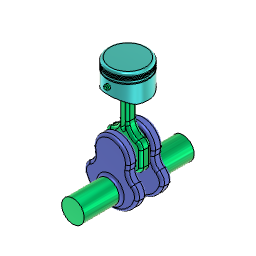
piston v2 (Autodesk Fusion 360 design; units mm, degrees)
Autodesk Fusion 360 part; units mm, degrees
sketch "Sketch1" plane through (0, 0, 0) normal (0, 0, 1) x (1, 0, 0) in component "Component"
  line L0 (100, 57.735) -> (0, 115.4701)
  line L1 (0, 115.4701) -> (-100, 57.735)
  line L2 (-100, 57.735) -> (-100, -57.735)
  line L3 (-100, -57.735) -> (0, -115.4701)
  line L4 (0, -115.4701) -> (100, -57.735)
  line L5 (100, -57.735) -> (100, 57.735)
  circle A0 centre (0, 0) radius 60
  constraint coincident A0.centre origin
extrude "Extrude1" add sketch "Sketch1" against normal blind 70 contours L0 L1 L2 L3 L4 L5 | A0 makes body 1 in component "Component"
extrude "Extrude2" add sketch "Sketch1" along normal blind 325 contours A0 bodies 1 in component "Component"
thread "Thread1" "ISO Metric profile 120.0 M120x6 6g" major diameter 119.62 minor diameter 112.7258 pitch 6 angle 60 resizes the face on face at (59.7018, -5.9741, 108.3333) from (0, 0, 75) to (0, 0, 325) on bodies 1 in component "Component"
sketch "Sketch1 (2)" plane through (0, 0, 0) normal (0, 1, 0) x (1, 0, 0) in component "piston"
  line L0 (0, -84) -> (0, -139)
  line L1 (0, -139) -> (40, -139)
  line L2 (40, -139) -> (40, -132)
  line L3 (40, -132) -> (36, -132)
  line L4 (36, -132) -> (36, -130)
  line L5 (36, -130) -> (40, -130)
  line L6 (40, -130) -> (40, -128)
  line L7 (40, -128) -> (36, -128)
  line L8 (36, -128) -> (36, -126)
  line L9 (36, -126) -> (40, -126)
  line L10 (40, -126) -> (40, -122)
  line L11 (40, -122) -> (36, -122)
  line L12 (36, -122) -> (36, -120)
  line L13 (36, -120) -> (40, -120)
  line L14 (40, -120) -> (40, -84)
  line L15 (40, -84) -> (0, -84)
  dimension "d7" = 40
  dimension "d8" = 4
  dimension "d9" = 4
  dimension "d10" = 7
  dimension "d11" = 2
  dimension "d12" = 2
  dimension "d13" = 2
  dimension "d14" = 4
  dimension "d15" = 2
  dimension "d16" = 36
  constraint vertical L0
  constraint perpendicular L0 L1
  constraint perpendicular L1 L2
  constraint perpendicular L2 L3
  constraint perpendicular L3 L4
  constraint perpendicular L4 L5
  constraint perpendicular L5 L6
  constraint perpendicular L6 L7
  constraint perpendicular L7 L8
  constraint perpendicular L6 L9
  constraint perpendicular L9 L10
  constraint perpendicular L10 L11
  constraint perpendicular L11 L12
  constraint perpendicular L12 L13
  constraint perpendicular L13 L14
  constraint perpendicular L0 L15
  constraint equal L3 L5
  constraint equal L5 L7
  constraint equal L7 L9
  constraint equal L11 L13
  measures "d7" distance of L0.end L1.end
  measures "d8" distance of L2.end L3.end
  measures "d9" distance of L10.end L11.end
  measures "d10" distance of L1.end L2.end
  measures "d11" distance of L3.end L4.end
  measures "d12" distance of L5.end L6.end
  measures "d13" distance of L7.end L8.end
  measures "d14" distance of L9.end L10.end
  measures "d15" distance of L11.end L12.end
  measures "d16" distance of L13.end L14.end
revolve "Revolve1" add sketch "Sketch1 (2)" angle 360 about axis through (0, 0, 1.75) along (0, 0, 1) separate body makes body 2 in component "piston"
move_body "Move1" bodies 2 to x (1, 0, 0) y (0, 1, 0) z (0, 0, 1) at (0, 0, -44) in component "piston"
sketch "Sketch2" plane through (0, 0, 0) normal (0, 1, 0) x (1, 0, 0) in component "piston"
  line L0 (0, 0) -> (0, -143.3697)
  line L1 (-40, -40) -> (40, -40)
  arc A0 (-35.5, -40) -> (35.5, -40) centre (0, 18.0125) ccw
  line L2 (-35.5, 0) -> (35.5, 0)
  line L3 (35.5, 0) -> (35.5, -40)
  line L4 (-35.5, -40) -> (-35.5, -36.7221)
  line L5 (-35.5, -36.7221) -> (-35.5, 0)
  point P0 (0, -50)
  point P1 (35.5, -40)
  point P2 (-35.5, -40)
  dimension "d18" = 10
  dimension "d19" = 4.5
  dimension "d20" = 4.5
  constraint coincident L0.start origin
  constraint vertical L0
  constraint coincident L0 P0
  constraint coincident L1 P1
  constraint coincident L1 P2
  constraint coincident P0 A0
  constraint coincident P1 A0.end
  constraint coincident P2 A0.start
  constraint perpendicular L0 L2
  constraint vertical L3
  constraint perpendicular L1 L4
  constraint perpendicular L2 L5
  measures "d18" distance of P0 L1
  measures "d19" distance of L1.end P1
  measures "d20" distance of L1.start P2
sketch "Sketch3" plane through (0, 0, 40) normal (0, 0, -1) x (1, 0, 0) in component "piston"
  circle A0 centre (0, 0) radius 40
  circle A1 centre (0, 0) radius 35.5
  dimension "d21" = 71
  constraint coincident A0.centre A1.centre
  measures "d21" diameter of A1
extrude "Extrude1'" cut sketch "Sketch3" against normal blind 33 contours A1 bodies 2 in component "piston"
extrude "Extrude2'" cut sketch "Sketch2" along normal mid plane 100 bodies 2 in component "piston"
sketch "Sketch4" plane through (0, 0, 0) normal (0, 1, 0) x (1, 0, 0) in component "piston"
  circle A0 centre (0, -64) radius 5
  line L0 (35.5, -40) -> (40, -40)
  dimension "d26" = 24
  measures "d26" distance of A0.centre L0
extrude "Extrude3" cut sketch "Sketch4" along normal mid plane 140 bodies 2 in component "piston"
sketch "Sketch5" plane through (0, 0, 0) normal (0, 1, 0) x (1, 0, 0) in component "piston"
  spline S0 degree 3 poles (-5, -64) (-5, -64.6285) (-4.8743, -65.2985) (-4.3638, -66.5302) (-3.9791, -67.092) (-3.092, -67.9791) (-2.5302, -68.3638) (-1.2985, -68.8743) (-0.6285, -69) (0.6285, -69) (1.2985, -68.8743) (2.5302, -68.3638) (3.092, -67.9791) (3.9791, -67.092) (4.3638, -66.5302) (4.8743, -65.2985) (5, -64.6285) (5, -63.3715) (4.8743, -62.7015) (4.3638, -61.4698) (3.9791, -60.908) (3.092, -60.0209) (2.5302, -59.6362) (1.2985, -59.1257) (0.6285, -59) (-0.6285, -59) (-1.2985, -59.1257) (-2.5302, -59.6362) (-3.092, -60.0209) (-3.9791, -60.908) (-4.3638, -61.4698) (-4.8743, -62.7015) (-5, -63.3715) (-5, -64) knots 0 0 0 0 0.188556 0.188556 0.377112 0.377112 0.565667 0.565667 0.754221 0.754221 0.942775 0.942775 1.13133 1.13133 1.319886 1.319886 1.508442 1.508442 1.696998 1.696998 1.885554 1.885554 2.074108 2.074108 2.262663 2.262663 2.451217 2.451217 2.639772 2.639772 2.828328 2.828328 3.016884 3.016884 3.016884 3.016884
  circle A0 centre (0, -64) radius 8.5
  line L0 (0, -64) -> (0, 59)
  circle A1 centre (0, 59) radius 23
  line L1 (36, 59) -> (36, 34)
  line L2 (0, 59) -> (36, 59)
  line L3 (8.5, -64) -> (8.5, 9)
  line L4 (36, 34) -> (33.5, 34)
  arc A2 (33.5, 34) -> (8.5, 9) centre (33.5, 9) ccw
  arc A3 (-8.5, 9) -> (-33.5, 34) centre (-33.5, 9) ccw
  line L5 (-8.5, -64) -> (-8.5, 9)
  line L6 (-36, 34) -> (-33.5, 34)
  line L7 (-36, 59) -> (-36, 34)
  line L8 (0, 59) -> (-36, 59)
  line L9 (4.6, 36.4647) -> (4.6, 59)
  line L10 (-4.6, 36.4647) -> (-4.6, 59)
  arc A4 (4.6, 24) -> (-4.6, 24) centre (0, 24) ccw
  line L11 (4.6, -64) -> (4.6, -56.8523)
  line L12 (4.6, -49) -> (4.6, 24)
  line L13 (-4.6, -64) -> (-4.6, -56.8523)
  line L14 (-4.6, -49) -> (-4.6, 24)
  arc A5 (-4.6, -49) -> (4.6, -49) centre (0, -49) ccw
  circle A6 centre (0, -64) radius 5
  line L15 (-36, 59) -> (-36, 89)
  line L16 (-36, 89) -> (36, 89)
  line L17 (36, 89) -> (36, 59)
  dimension "d29" = 17
  dimension "d30" = 123
  dimension "d31" = 46
  dimension "d32" = 36
  dimension "d33" = 25
  dimension "d34" = 25
  dimension "d37" = 9.2
  dimension "d38" = 15
  dimension "d39" = 9.2
  dimension "d40" = 35
  dimension "d41" = 10
  dimension "d42" = 30
  constraint coincident A0.centre L0.start
  constraint vertical L0
  constraint coincident L0.end A1.centre
  constraint vertical L1
  constraint perpendicular L1 L2
  constraint coincident A0 L3.start
  constraint perpendicular L2 L3
  constraint perpendicular L3 L4
  constraint tangent L3 A2
  constraint tangent L4 A2
  constraint symmetric L0 L1.end L6.start
  constraint symmetric L0 A1.centre L2.start
  constraint symmetric L0 L1.start L7.start
  constraint symmetric L0 L3.start L5.start
  constraint symmetric L0 L3.end A3.start
  constraint symmetric L0 L4.end A3.end
  constraint symmetric L0 A2 A3
  constraint coincident L0 A5.centre
  constraint coincident L0 A4.centre
  constraint tangent A4 L11
  constraint parallel L0 L11
  constraint coincident A1 L9.start
  constraint collinear L9 L11
  constraint parallel L0 L13
  constraint coincident A1 L10.start
  constraint collinear L10 L13
  constraint coincident A0 L11.end
  constraint collinear L11 L12
  constraint coincident A0 L13.end
  constraint collinear L13 L14
  constraint concentric A0 A6
  constraint perpendicular L8 L15
  constraint perpendicular L7 L16
  constraint vertical L17
  measures "d29" diameter of A0
  measures "d30" distance of A0.centre L0.end
  measures "d31" diameter of A1
  measures "d32" distance of L0.end L1
  measures "d33" distance of L1.end L1.start
  measures "d34" radius of A2
  measures "d37" diameter of A5
  measures "d38" distance of A0.centre A5.centre
  measures "d39" diameter of A4
  measures "d40" distance of L0.end A4.centre
  measures "d41" diameter of A6
  measures "d42" distance of L7.start L15.end
extrude "Extrude1''" add sketch "Sketch5" along normal mid plane 20 separate body contours S0 A0 L11 L13 A6 | S0 A0 L0 L13 A6 | S0 A0 L0 L11 A6 | A0 L0 A1 A3 L5 L6 L7 L8 A4 L14 A5 | A0 L0 A1 L1 L2 L3 L4 A2 A4 L12 A5 | A1 L2 L8 L15 L16 L17 makes body 3 in component "connecting rod"
fillet "Fillet1" radius 13 2 edges at (36, 0, -34) (-36, 0, -34) on bodies 3 in component "connecting rod"
fillet "Fillet2" radius 13 2 edges at (36, 0, -89) (-36, 0, -89) on bodies 3 in component "connecting rod"
sketch "Sketch1 (3)" plane through (0, 0, 0) normal (0, 1, 0) x (1, 0, 0)
  line L0 (35, 59) -> (-35, 59)
  line L1 (35, 59) -> (33.5793, 48.8838)
  line L2 (-35, 59) -> (-33.5793, 48.8838)
  line L3 (54.9124, 26.1024) -> (53.385, 26.1024)
  line L4 (-53.385, 26.1024) -> (-54.9124, 26.1024)
  arc A0 (-54.9124, 26.1024) -> (54.9124, 26.1024) centre (0, 23) ccw
  arc A1 (35, 59) -> (-35, 59) centre (0, 59) ccw
  arc A2 (-53.385, 26.1024) -> (-33.5793, 48.8838) centre (-53.385, 46.1024) ccw
  arc A3 (33.5793, 48.8838) -> (53.385, 26.1024) centre (53.385, 46.1024) ccw
  circle A4 centre (0, 1) radius 22.5
  dimension "d54" = 110
  dimension "d55" = 36
  dimension "d56" = 70
  dimension "d57" = 20
  dimension "d58" = 45
  dimension "d59" = 22
  constraint collinear L3 L4
  constraint tangent L2 A2
  constraint tangent L4 A2
  constraint tangent L1 A3
  constraint tangent L3 A3
  constraint equal A2 A3
  constraint coincident L0 A1.centre
  constraint horizontal L0
  measures "d54" diameter of A0
  measures "d55" distance of A0.centre A1.centre
  measures "d56" diameter of A1
  measures "d57" radius of A2
  measures "d58" diameter of A4
  measures "d59" distance of A0.centre A4.centre
extrude "Extrude1'''" add sketch "Sketch1 (3)" along normal blind 20 from surface at 15 separate body makes body 4 in component "crank shaft"
sketch "Sketch2 (2)" plane through (0, 35, 0) normal (0, 1, 0) x (-1, 0, 0)
  circle A0 centre (0, -1) radius 22.5
  arc A1 (-35, -59) -> (35, -59) centre (0, -59) ccw
  line L0 (35, -59) -> (33.5793, -48.8838)
  arc A2 (53.385, -26.1024) -> (33.5793, -48.8838) centre (53.385, -46.1024) ccw
  line L1 (53.385, -26.1024) -> (54.9124, -26.1024)
  arc A3 (54.9124, -26.1024) -> (-54.9124, -26.1024) centre (0, -23) ccw
  line L2 (-54.9124, -26.1024) -> (-53.385, -26.1024)
  arc A4 (-33.5793, -48.8838) -> (-53.385, -26.1024) centre (-53.385, -46.1024) ccw
  line L3 (-33.5793, -48.8838) -> (-35, -59)
extrude "Extrude2''" add sketch "Sketch2 (2)" along normal blind 75 and the other way blind 20 contours A0 bodies 4 in component "crank shaft"
sketch "Sketch3 (2)" plane through (0, -32, 0) normal (0, -1, 0) x (1, 0, 0)
  circle A0 centre (0, -1) radius 22.5
  arc A1 (15.85, -75.6667) -> (23, -59) centre (0, -59) ccw
  line L0 (23, -59) -> (23, -48)
  arc A2 (48, -23) -> (23, -48) centre (48, -48) ccw
  line L1 (48, -23) -> (55, -23)
  arc A3 (55, -23) -> (-55, -23) centre (0, -23) ccw
  line L2 (-55, -23) -> (-48, -23)
  arc A4 (-23, -48) -> (-48, -23) centre (-48, -48) ccw
  line L3 (-23, -48) -> (-23, -59)
  arc A5 (-23, -59) -> (-15.85, -75.6667) centre (0, -59) ccw
  arc A6 (-15.85, -75.6667) -> (15.85, -75.6667) centre (0, -23) ccw
sketch "Sketch4 (2)" plane through (0, 0, 0) normal (0, 1, 0) x (1, 0, 0)
mirror "Mirror1" about plane through (0, 0, 0) normal (0, 1, 0) of bodies 4 makes body 5 in component "crank shaft"
extrude "Extrude5" add sketch "Sketch5" along normal mid plane 40 contours L0 A1 L8 L10 | L0 A1 L2 L9 | A1 L2 L8 | A1 L8 L10 | A1 L2 L9 bodies 4 5 in component "crank shaft"
fillet "Fillet1'" radius 20 4 edges at (54.9124, -25, -26.1024) (54.9124, 25, -26.1024) (-54.9124, -25, -26.1024) (-54.9124, 25, -26.1024) on bodies 4 5 in component "crank shaft"
fillet "Fillet2'" radius 5 4 faces at (-0.5605, -35, -40.4016) (-31.301, 15, -19.6844) (-31.301, -15, -19.6844) (-0.5605, 35, -40.4016) on bodies 4 in component "crank shaft"
fillet "Fillet3" radius 5 24 edges at (0, -10, 72.5) (-8.5, -10, 27.5) (-13.5288, -10, -24.0383) (-33.385, -10, -37.7006) (-36, -10, -60.7603) (-32.1924, -10, -85.1924) (0, -10, -89) (32.1924, -10, -85.1924) (36, -10, -60.7603) (33.385, -10, -37.7006) (13.5288, -10, -24.0383) (8.5, -10, 27.5) (13.5288, 10, -24.0383) (33.385, 10, -37.7006) (36, 10, -60.7603) (32.1924, 10, -85.1924) (0, 10, -89) (-32.1924, 10, -85.1924) (-36, 10, -60.7603) (-33.385, 10, -37.7006) (-13.5288, 10, -24.0383) (-8.5, 10, 27.5) (0, 10, 72.5) (8.5, 10, 27.5) on bodies 3 in component "connecting rod"
sketch "Sketch5 (2)" plane through (0, 0, 0) normal (0, 1, 0) x (1, 0, 0)
  spline S0 degree 3 poles (-5, -64) (-5, -64.6285) (-4.8743, -65.2985) (-4.3638, -66.5302) (-3.9791, -67.092) (-3.092, -67.9791) (-2.5302, -68.3638) (-1.2985, -68.8743) (-0.6285, -69) (0.6285, -69) (1.2985, -68.8743) (2.5302, -68.3638) (3.092, -67.9791) (3.9791, -67.092) (4.3638, -66.5302) (4.8743, -65.2985) (5, -64.6285) (5, -63.3715) (4.8743, -62.7015) (4.3638, -61.4698) (3.9791, -60.908) (3.092, -60.0209) (2.5302, -59.6362) (1.2985, -59.1257) (0.6285, -59) (-0.6285, -59) (-1.2985, -59.1257) (-2.5302, -59.6362) (-3.092, -60.0209) (-3.9791, -60.908) (-4.3638, -61.4698) (-4.8743, -62.7015) (-5, -63.3715) (-5, -64) knots 0 0 0 0 0.188556 0.188556 0.377112 0.377112 0.565667 0.565667 0.754221 0.754221 0.942775 0.942775 1.13133 1.13133 1.319886 1.319886 1.508442 1.508442 1.696998 1.696998 1.885554 1.885554 2.074108 2.074108 2.262663 2.262663 2.451217 2.451217 2.639772 2.639772 2.828328 2.828328 3.016884 3.016884 3.016884 3.016884
extrude "Extrude1''''" add sketch "Sketch5 (2)" along normal mid plane 90 separate body makes body 6 in component "piston pin"
fillet "Fillet1''" radius 2 2 faces at (-0.8987, -45, 62.6285) (-0.8987, 45, 62.6285) on bodies 6 in component "piston pin"
sketch "Sketch6" plane through (0, -110, 0) normal (0, -1, 0) x (1, 0, 0)
  circle A0 centre (0, -1) radius 22.5
  circle A1 centre (0, 0) radius 55.9017
  constraint coincident A1.centre origin
extrude "Extrude1'''''" add sketch "Sketch6" along normal blind 40 separate body makes body 7 in component "Component'"
fillet "Fillet2''" radius 5 1 faces at (7.7208, -6.4944, 95) on bodies 2 in component "piston"
sketch "Sketch7" plane through (0, 0, 95) normal (0, 0, 1) x (-1, 0, 0)
  circle A0 centre (0, 0.0021) radius 35
  circle A1 centre (0, 0) radius 123.9303
  constraint coincident A1.centre origin
extrude "Extrude1''''''" add sketch "Sketch7" along normal blind 70 separate body makes body 8 in component "Component''"
move_body "Move1'" bodies 6 to x (1, 0, 0) y (0, 1, 0) z (0, 0, 1) at (0, 0, 116) in component "piston pin"
component "Component" placed x (1, 0, 0) y (0, 1, 0) z (0, 0, 1) at (0, 0, 0)
component "piston" placed x (1, 0, 0) y (0, 1, 0) z (0, 0, 1) at (0, -0.0021, 116)
component "crank shaft" placed x (-1, 0, 0) y (0, 1, 0) z (0, 0, -1) at (0, 0, -2)
component "piston pin" placed x (1, 0, 0) y (0, 1, 0) z (0, 0, 1) at (0, 0, 0)
component "Component'" placed x (1, 0, 0) y (0, 1, 0) z (0, 0, 1) at (0, 0, 0)
component "connecting rod" placed x (1, 0, 0) y (0, 1, 0) z (0, 0, 1) at (0, 0, 116)
component "Component''" placed x (1, 0, 0) y (0, 1, 0) z (0, 0, 1) at (0, 0, 0)
